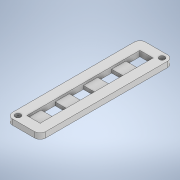
# Autodesk Inventor part: open_side
Saved by Autodesk Inventor 2020 (Build 240168000, 168)
## iProperties
Created: 2019-05-06
Part Number: open_side
Material: Generic
Document SubType Name: Modeling
Designer: erwin
Density: 1 g/cm^3
Appearance: Default
Author: erwin
Autodesk Inventor part; units mm, degrees
ref_plane "YZ Plane" through (0, 0, 0) normal (1, 0, 0) x (0, 1, 0)
ref_plane "XZ Plane" through (0, 0, 0) normal (0, 1, 0) x (-1, 0, 0)
ref_plane "XY Plane" through (0, 0, 0) normal (0, 0, 1) x (1, 0, 0)
sketch "Sketch1" plane through (0, 0, 0) normal (0, 1, 0) x (-1, 0, 0)
  line L0 (15, 60) -> (-15, 60)
  line L1 (-15, 60) -> (-15, -60)
  line L2 (-15, -60) -> (15, -60)
  line L3 (15, -60) -> (15, 60)
  line L4 (15, 60) -> (-15, -60) construction
  line L5 (-15, 60) -> (15, -60) construction
  point P0 (0, 0)
  dimension "d0" = 30
  dimension "d1" = 120
  constraints: 12 end point, 2 midpoint, 2 parallel, 1 horizontal, 1 perpendicular
  measures "d0" distance of L2.end L1.end
  measures "d1" distance of L1.end L0.end
extrude "Extrusion1" add sketch "Sketch1" along normal blind 5
sketch "Sketch2" plane through (0, 5, 0) normal (0, 1, 0) x (1, 0, 0)
  line L0 (-6, -51) -> (6, -51)
  line L1 (6, -51) -> (6, 51)
  line L2 (6, 51) -> (-6, 51)
  line L3 (-6, 51) -> (-6, -51)
  line L4 (-6, -51) -> (6, 51) construction
  line L5 (6, -51) -> (-6, 51) construction
  line L6 (-15, 60) -> (-15, -60) projected
  point P0 (0, 0)
  point P1 (0, 0)
  point P2 (0, 0)
  dimension "d4" = 12
  dimension "d5" = 102
  constraints: 12 end point, 3 midpoint, 2 parallel, 1 coincident, 1 horizontal, 1 perpendicular
  measures "d4" distance of L2.end L1.end
  measures "d5" distance of L1.end L0.end
extrude "Extrusion2" cut sketch "Sketch2" against normal blind 2
sketch "Sketch3" plane through (0, 3, 0) normal (0, 1, 0) x (1, 0, 0)
  line L0 (-6, -51) -> (-6, 51) projected
  line L1 (6, 51) -> (6, -51) projected
  line L2 (-6, -38.25) -> (6, -38.25)
  line L3 (6, -38.25) -> (6, -25.5)
  line L4 (6, -25.5) -> (-6, -25.5)
  line L5 (-6, -25.5) -> (-6, -38.25)
  line L6 (6, -51) -> (-6, -51) projected
  line L7 (-6, -12.75) -> (6, -12.75)
  line L8 (6, -12.75) -> (6, 0)
  line L9 (6, 0) -> (-6, 0)
  line L10 (-6, 0) -> (-6, -12.75)
  line L11 (-6, 12.75) -> (6, 12.75)
  line L12 (6, 12.75) -> (6, 25.5)
  line L13 (6, 25.5) -> (-6, 25.5)
  line L14 (-6, 25.5) -> (-6, 12.75)
  line L15 (-6, 38.25) -> (6, 38.25)
  line L16 (6, 38.25) -> (6, 51)
  line L17 (6, 51) -> (-6, 51)
  line L18 (-6, 51) -> (-6, 38.25)
  point P0 (0, 0)
  point P1 (-6, 51)
  point P2 (-6, 38.25)
  point P3 (6, 38.25)
  point P4 (6, 25.5)
  point P5 (-6, 25.5)
  point P6 (-6, 12.75)
  point P7 (6, 12.75)
  point P8 (6, 0)
  point P9 (-6, 0)
  point P10 (-6, -12.75)
  point P11 (6, -12.75)
  point P12 (-6, -25.5)
  point P13 (6, -38.25)
  dimension "d9" = 12.75
  dimension "d10" = 12.75
  dimension "d13" = 25.5
  constraints: 32 end point, 2 parallel, 2 point on line, 1 horizontal, 1 perpendicular, 1 vertical, 24 other
  measures "d9" distance between parallel lines of L2 L4
  measures "d10" distance between parallel lines of L6 L2
  measures "d13" distance of L2.start L7.start
extrude "Extrusion3" cut sketch "Sketch3" against normal through all contours L0 L4 L1 L2 | L0 L9 L1 L7 | L0 L13 L1 L11 | L0 L17 L1 L15
fillet "Fillet1" radius 5 4 edges at (15, 2.5, 60) (15, 2.5, -60) (-15, 2.5, -60) (-15, 2.5, 60)
sketch "Sketch4" plane through (0, 5, 0) normal (0, 1, 0) x (1, 0, 0)
  arc A0 (-15, -55) -> (-10, -60) centre (-10, -55) ccw projected
  arc A1 (15, 55) -> (10, 60) centre (10, 55) ccw projected
  point P0 (0, 0)
  constraints: 2 coincident
hole "Hole1" at (-10, 5, 55) at (10, 5, -55) direction (0, -1, 0) diameter 3 end through all counterbore diameter 5 counterbore depth 2
equation "\"d9\" = d10"
equation "\"d10\" = 0.125 * d5"
equation "\"d13\" = 2 * d10"
body "Solid1"
